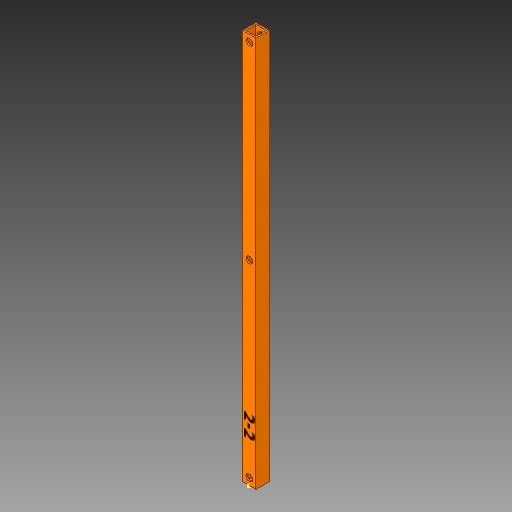
# Autodesk Inventor part: 2018 Bar2_2
Saved by Autodesk Inventor 2018 (Build 220112000, 112)
## iProperties
Created: 2018-01-17
Part Number: 2018 Bar2_2
Material: Generic
Document SubType Name: Modeling
Designer: Apple
Density: 1 g/cm^3
Appearance: Default
Author: Apple
Autodesk Inventor part; units mm, degrees
ref_plane "YZ Plane" through (0, 0, 0) normal (1, 0, 0) x (0, 1, 0)
ref_plane "XZ Plane" through (0, 0, 0) normal (0, 1, 0) x (-1, 0, 0)
ref_plane "XY Plane" through (0, 0, 0) normal (0, 0, 1) x (1, 0, 0)
sketch "Sketch1" plane through (0, 0, 0) normal (0, 1, 0) x (-1, 0, 0)
  line L0 (12.7, 12.7) -> (-12.7, 12.7)
  line L1 (-12.7, 12.7) -> (-12.7, -12.7)
  line L2 (-12.7, -12.7) -> (12.7, -12.7)
  line L3 (12.7, -12.7) -> (12.7, 12.7)
  line L4 (-9.525, 9.525) -> (9.525, 9.525)
  line L5 (9.525, 9.525) -> (9.525, -9.525)
  line L6 (9.525, -9.525) -> (-9.525, -9.525)
  line L7 (-9.525, -9.525) -> (-9.525, 9.525)
  point P0 (0, 0)
  point P1 (12.7, 0)
  point P2 (0, -12.7)
  dimension "d0" = 25.4
  dimension "d1" = 25.4
  dimension "d2" = 3.175
  constraints: 16 end point, 4 parallel, 2 midpoint, 2 perpendicular, 1 horizontal, 1 horizontal alignment, 1 vertical alignment, 3 other
  measures "d0" distance of L2.end L0.start
  measures "d1" distance of L1.end L2.end
  measures "d2" distance between parallel lines of L4 L0
extrude "Extrusion1" add sketch "Sketch1" along normal blind 736.6
sketch "Sketch2" plane through (-12.7, 0, 12.7) normal (0, 0, 1) x (1, 0, 0)
  line L0 (0, 736.6) -> (25.4, 736.6) projected
  line L1 (0, 0) -> (25.4, 0) projected
  point P0 (12.7, 0)
  point P1 (12.7, 12.7)
  point P2 (12.7, 723.9)
  point P3 (12.7, 368.3)
  dimension "d5" = 12.7
  dimension "d6" = 12.7
  dimension "d7" = 368.3
  measures "d5" distance from line of point (12.7, 723.9) L0
  measures "d6" distance from line of L1 point (12.7, 12.7)
  measures "d7" distance from line of L1 point (12.7, 368.3)
hole "Hole1" at (0, 12.7, 12.7) at (0, 723.9, 12.7) at (0, 368.3, 12.7) direction (0, 0, -1) diameter 12.7 end through all
sketch "Sketch3" plane through (-12.7, 0, 12.7) normal (0, 0, 1) x (1, 0, 0)
  line L0 (22.3523, 119.127) -> (22.3523, 87.2161) construction
  line L1 (22.3523, 87.2161) -> (-37.8014, 87.2161) construction
  line L2 (-37.8014, 87.2161) -> (-37.8014, 119.127) construction
  line L3 (-37.8014, 119.127) -> (22.3523, 119.127) construction
  point P0 (12.7, 0)
  constraints: 2 other
equation "\"d0\" = Tube_size"
equation "\"d1\" = Tube_size"
equation "\"d2\" = Wall_Thickness"
equation "\"d3\" = Bar2_2_Length"
equation "\"d5\" = Uper_Pivit_Offset_FromEdge"
equation "\"d6\" = Lower_Pivit_Offset_FromEdge"
equation "\"d7\" = Bar2_2_Center_Pivit_Offset_FromEdge"
equation "\"d8\" = Pin_Size"
equation "\"Bar1_1_Length\" = 736.6"
equation "\"Lower_Pivit_Offset_FromEdge\" = 12.7"
equation "\"Uper_Pivit_Offset_FromEdge\" = 12.7"
equation "\"Bar1_1_Center_Pivit_Offset_FromEdge\" = 368.3"
equation "\"Bar1_2_Length\" = 736.6"
equation "\"Bar2_1_Length\" = 736.6"
equation "\"Bar2_2_Length\" = 736.6"
equation "\"Bar3_1_Length\" = 736.6"
equation "\"Bar3_2_Length\" = 736.6"
equation "\"Tube_size\" = 25.4"
equation "\"Wall_Thickness\" = 3.175"
equation "\"Bar1_2_Center_Pivit_Offset_FromEdge\" = 368.3"
equation "\"Bar2_1_Center_Pivit_Offset_FromEdge\" = 368.3"
equation "\"Bar2_2_Center_Pivit_Offset_FromEdge\" = 368.3"
equation "\"Bar3_1_Center_Pivit_Offset_FromEdge\" = 368.3"
equation "\"Bar4_2_Center_Pivit_Offset_FromEdge\" = 355.6"
equation "\"Pin_Size\" = 12.7"
equation "\"Bar3_2_Center_Pivit_Offset_FromEdge\" = 368.3"
body "Solid1"
